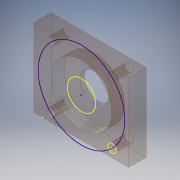
# Autodesk Inventor part: polycarb_front
Saved by Autodesk Inventor 2017 (Build 210142000, 142)
## iProperties
Created: 2017-08-10
Part Number: polycarb_front
Material: Polycarbonate, Smoke
Document SubType Name: Modeling
Designer: Kai
Density: 1.2 g/cm^3
Appearance: Polycarbonate - Smoked
Author: Kai
Autodesk Inventor part; units mm, degrees
ref_plane "YZ Plane" through (0, 0, 0) normal (1, 0, 0) x (0, 1, 0)
ref_plane "XZ Plane" through (0, 0, 0) normal (0, 1, 0) x (-1, 0, 0)
ref_plane "XY Plane" through (0, 0, 0) normal (0, 0, 1) x (1, 0, 0)
sketch "Sketch1" plane through (0, 0, 0) normal (0, 0, 1) x (1, 0, 0)
  line L0 (0, 0) -> (57.15, 0)
  line L1 (57.15, 0) -> (57.15, 57.15)
  line L2 (57.15, 57.15) -> (0, 57.15)
  line L3 (0, 57.15) -> (0, 0)
  line L4 (0, 57.15) -> (57.15, 0) construction
  circle A0 centre (28.575, 28.575) radius 31.825 construction
  line L5 (0, 0) -> (57.15, 57.15) construction
  circle A1 centre (6.0713, 51.0787) radius 3.1
  circle A2 centre (6.0713, 6.0713) radius 3.1
  circle A3 centre (51.0787, 6.0713) radius 3.1
  circle A4 centre (51.0787, 51.0787) radius 3.1
  circle A5 centre (28.575, 28.575) radius 11.1125
  dimension "d2" = 63.65
  dimension "d0" = 57.15
  dimension "d1" = 57.15
  dimension "d3" = 6.2
  dimension "d6" = 360
  dimension "d10" = 22.225
  constraints: 12 end point, 5 centre point, 2 parallel, 1 coincident, 1 horizontal, 1 midpoint, 1 perpendicular, 1 point on line, 12 other
  measures "d0" distance of L2.end L1.end
  measures "d1" distance of L1.end L0.end
  measures "d3" diameter of A1
  measures "d10" diameter of A5
extrude "Extrusion1" add sketch "Sketch1" along normal blind 12.7 contours L3 L2 L1 L0 | A5
sketch "Sketch2" plane through (0, 0, 12.7) normal (0, 0, 1) x (1, 0, 0)
  circle A0 centre (28.575, 28.575) radius 10.5
  line L0 (57.15, 57.15) -> (0, 57.15) projected
  line L1 (57.15, 0) -> (57.15, 57.15) projected
  point P0 (0, 0)
  dimension "d11" = 21
  dimension "d12" = 28.575
  dimension "d13" = 28.575
  constraints: 1 centre point
  measures "d11" diameter of A0
  measures "d12" distance from line of L0 A0.centre
  measures "d13" distance from line of L1 A0.centre
extrude "Extrusion2" cut sketch "Sketch2" against normal blind 25.4
sketch "Sketch3" plane through (0, 0, 12.7) normal (0, 0, 1) x (1, 0, 0)
  circle A0 centre (28.575, 28.575) radius 10.5 projected
  circle A1 centre (28.575, 28.575) radius 22.225
  point P0 (0, 0)
  dimension "d16" = 44.45
  constraints: 1 centre point, 1 coincident
  measures "d16" diameter of A1
extrude "Extrusion3" cut sketch "Sketch3" against normal blind 9.525
sketch "Sketch4" plane through (0, 0, 12.7) normal (0, 0, 1) x (1, 0, 0)
  line L0 (0, 57.15) -> (0, 0) projected
  line L1 (0, 57.15) -> (-6.35, 57.15)
  line L2 (-6.35, 57.15) -> (-6.35, 0)
  line L3 (-6.35, 0) -> (0, 0)
  line L4 (0, 0) -> (0, 57.15)
  line L5 (57.15, 0) -> (57.15, 57.15) projected
  line L6 (57.15, 57.15) -> (63.5, 57.15)
  line L7 (63.5, 57.15) -> (63.5, 0)
  line L8 (63.5, 0) -> (57.15, 0)
  line L9 (57.15, 0) -> (57.15, 57.15)
  dimension "d19" = 6.35
  dimension "d20" = 6.35
  constraints: 16 end point, 4 parallel, 2 horizontal, 2 perpendicular, 1 point on line
  measures "d19" distance of L3.end L2.end
  measures "d20" distance of L7.end L8.end
extrude "Extrusion4" add sketch "Sketch4" against normal up to surface (12.7 mm away)
sketch "Sketch5" plane through (0, 0, 12.7) normal (0, 0, 1) x (1, 0, 0)
  circle A0 centre (28.575, 28.575) radius 10.5 projected
  circle A1 centre (51.0787, 6.0713) radius 3.1 projected
  circle A2 centre (28.575, 28.575) radius 31.825
  point P0 (0, 0)
  constraints: 1 coincident, 3 other
body "Solid1"
